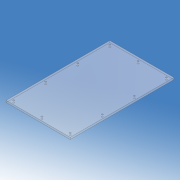
# Autodesk Inventor part: NASA-20-EBOX-B-01
Saved by Autodesk Inventor 2020 (Build 240168000, 168)
## iProperties
Company: Kent State Robotics
Created: 2019-09-23
Part Number: NASA-20-EBOX-B-01
Material: Polycarbonate, Clear
Document SubType Name: Modeling
Designer: Michael Parker
Density: 1.2 g/cm^3
Appearance: Polycarbonate - Clear
Description: Electronics box bottom
Mass: 573.838 g
Surface Area: 1584.89 cm^2
Volume: 478.199 cm^3
Author: Michael Parker
Title: Electronics Box Bottom Panel
Autodesk Inventor part; units mm, degrees
ref_plane "YZ Plane" through (0, 0, 0) normal (1, 0, 0) x (0, 1, 0)
ref_plane "XZ Plane" through (0, 0, 0) normal (0, 1, 0) x (-1, 0, 0)
ref_plane "XY Plane" through (0, 0, 0) normal (0, 0, 1) x (1, 0, 0)
sketch "Sketch1" plane through (0, 0, 0) normal (0, 1, 0) x (-1, 0, 0)
  line L0 (107.95, -174.625) -> (-107.95, -174.625)
  line L1 (-107.95, -174.625) -> (-107.95, 174.625)
  line L2 (-107.95, 174.625) -> (107.95, 174.625)
  line L3 (107.95, 174.625) -> (107.95, -174.625)
  line L4 (107.95, -174.625) -> (-107.95, 174.625) construction
  line L5 (-107.95, -174.625) -> (107.95, 174.625) construction
  point P0 (0, 0)
  dimension "d0" = 215.9
  dimension "d1" = 349.25
  constraints: 12 end point, 2 midpoint, 2 parallel, 1 horizontal, 1 perpendicular
  measures "d0" distance of L1.end L2.end
  measures "d1" distance of L0.end L1.end
extrude "Extrusion1" add sketch "Sketch1" along normal blind 6.35
sketch "Sketch2" plane through (0, 0, 0) normal (0, -1, 0) x (1, 0, 0)
  circle A0 centre (-95.25, 53.975) radius 1.75 projected
  circle A1 centre (0, 161.925) radius 1.75 projected
  circle A2 centre (95.25, 53.975) radius 1.75 projected
  circle A3 centre (95.25, 161.925) radius 1.75 projected
  circle A4 centre (-95.25, 161.925) radius 1.75 projected
  circle A5 centre (-95.25, -161.925) radius 1.75 projected
  circle A6 centre (95.25, -161.925) radius 1.75 projected
  circle A7 centre (95.25, -53.975) radius 1.75 projected
  circle A8 centre (0, -161.925) radius 1.75 projected
  circle A9 centre (-95.25, -53.975) radius 1.75 projected
  circle A10 centre (-65.0875, -144.0656) radius 1.75 projected
  circle A11 centre (65.0875, -144.0656) radius 1.75 projected
  circle A12 centre (49.2125, -144.0656) radius 1.75 projected
  circle A13 centre (-49.2125, -144.0656) radius 1.75 projected
  line L0 (-82.55, -136.525) -> (82.55, -136.525) projected
  line L1 (82.55, -136.525) -> (82.55, 136.525) projected
  line L2 (82.55, 136.525) -> (-82.55, 136.525) projected
  line L3 (-82.55, 136.525) -> (-82.55, -136.525) projected
  line L4 (107.95, -174.625) -> (-107.95, -174.625) projected
  line L5 (-107.95, -174.625) -> (-107.95, 174.625) projected
  line L6 (-107.95, 174.625) -> (107.95, 174.625) projected
  line L7 (107.95, 174.625) -> (107.95, -174.625) projected
  point P0 (0, 0)
hole "Hole1" at (95.25, 0, -161.925) at (0, 0, -161.925) at (-95.25, 0, -161.925) at (-95.25, 0, -53.975) at (-95.25, 0, 53.975) at (-95.25, 0, 161.925) at (0, 0, 161.925) at (95.25, 0, 161.925) at (95.25, 0, 53.975) at (95.25, 0, -53.975) direction (0, 1, 0) diameter 5.5 end through all
sketch "Electronics Area" plane through (0, 6.35, 0) normal (0, 1, 0) x (1, 0, 0)
  line L0 (-88.9, -155.575) -> (88.392, -155.575) projected
  line L1 (-88.9, 174.625) -> (-88.9, -485.775) projected
  line L2 (88.392, 155.575) -> (-88.9, 155.575) projected
  line L3 (88.9, 174.625) -> (88.9, -485.775) projected
  line L4 (88.9, 155.575) -> (-88.9, 155.575)
  line L5 (-88.9, 155.575) -> (-88.9, -155.575)
  line L6 (-88.9, -155.575) -> (88.9, -155.575)
  line L7 (88.9, -155.575) -> (88.9, 155.575)
  line L8 (76.2, 142.875) -> (-76.2, 142.875)
  line L9 (-76.2, 142.875) -> (-76.2, -142.875)
  line L10 (-76.2, -142.875) -> (76.2, -142.875)
  line L11 (76.2, -142.875) -> (76.2, 142.875)
  point P0 (0, 0)
  dimension "d11" = 12.7
  constraints: 16 end point, 4 parallel, 2 perpendicular, 2 point on line, 1 horizontal, 3 other
  measures "d11" distance between parallel lines of L7 L11
body "Solid1"
